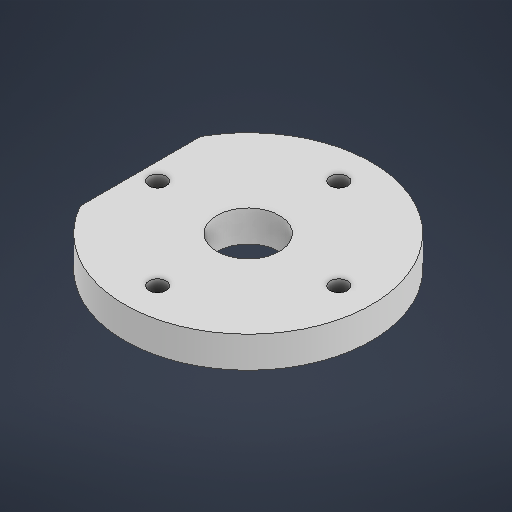
# Autodesk Inventor part: Adapter Plate
Saved by Autodesk Inventor 2025 (Build 290162000, 162)
## iProperties
Created: 2024-09-13
Part Number: Adapter Plate
Material: Generic
Document SubType Name: Modeling
Designer: mayhe
Density: 1 g/cm^3
Appearance: Default
Author: mayhe
Autodesk Inventor part; units mm, degrees
ref_plane "YZ Plane" through (0, 0, 0) normal (1, 0, 0) x (0, 1, 0)
ref_plane "XZ Plane" through (0, 0, 0) normal (0, 1, 0) x (-1, 0, 0)
ref_plane "XY Plane" through (0, 0, 0) normal (0, 0, 1) x (1, 0, 0)
sketch "Sketch1" plane through (0, 0, 0) normal (0, 1, 0) x (-1, 0, 0)
  circle A0 centre (0, 0) radius 39.5
  circle A1 centre (0, 0) radius 10
  circle A2 centre (0, 0) radius 29
  circle A3 centre (29, 0) radius 2.75
  circle A4 centre (0, 29) radius 2.75
  circle A5 centre (-29, 0) radius 2.75
  circle A6 centre (0, -29) radius 2.75
  dimension "d2" = 58
  dimension "d0" = 79
  dimension "d1" = 20
  dimension "d3" = 5.5
  dimension "d6" = 360
  constraints: 6 centre point, 3 coincident, 1 horizontal alignment, 11 other
  measures "d0" diameter of A0
  measures "d1" diameter of A1
  measures "d3" diameter of A3
extrude "Extrusion1" add sketch "Sketch1" along normal blind 10 contours A0 | A3 A2 A6 A5 A4
sketch "Sketch2" plane through (0, 0, 0) normal (0, -1, 0) x (1, 0, 0)
  circle A0 centre (0, -29) radius 2.75 projected
  circle A1 centre (0, 0) radius 29
  circle A2 centre (29, 0) radius 2.75 projected
  circle A3 centre (29, 0) radius 4
  circle A4 centre (0, 29) radius 4
  circle A5 centre (-29, 0) radius 4
  circle A6 centre (0, -29) radius 4
  line L0 (25, 2.3094) -> (29, 4.6188)
  line L1 (29, 4.6188) -> (33, 2.3094)
  line L2 (33, 2.3094) -> (33, -2.3094)
  line L3 (33, -2.3094) -> (29, -4.6188)
  line L4 (29, -4.6188) -> (25, -2.3094)
  line L5 (25, -2.3094) -> (25, 2.3094)
  line L6 (-4, -26.6906) -> (0, -24.3812)
  line L7 (0, -24.3812) -> (4, -26.6906)
  line L8 (4, -26.6906) -> (4, -31.3094)
  line L9 (4, -31.3094) -> (0, -33.6188)
  line L10 (0, -33.6188) -> (-4, -31.3094)
  line L11 (-4, -31.3094) -> (-4, -26.6906)
  line L12 (-33, 2.3094) -> (-29, 4.6188)
  line L13 (-29, 4.6188) -> (-25, 2.3094)
  line L14 (-25, 2.3094) -> (-25, -2.3094)
  line L15 (-25, -2.3094) -> (-29, -4.6188)
  line L16 (-29, -4.6188) -> (-33, -2.3094)
  line L17 (-33, -2.3094) -> (-33, 2.3094)
  line L18 (-4, 31.3094) -> (0, 33.6188)
  line L19 (0, 33.6188) -> (4, 31.3094)
  line L20 (4, 31.3094) -> (4, 26.6906)
  line L21 (4, 26.6906) -> (0, 24.3812)
  line L22 (0, 24.3812) -> (-4, 26.6906)
  line L23 (-4, 26.6906) -> (-4, 31.3094)
  circle A7 centre (0, 29) radius 2.75
  circle A8 centre (-29, 0) radius 2.75
  point P0 (25, 0)
  point P1 (-4, -29)
  point P2 (-33, 0)
  point P3 (-4, 29)
  dimension "d10" = 8
  dimension "d13" = 360
  constraints: 48 end point, 8 coincident, 4 horizontal alignment, 4 midpoint, 2 centre point, 1 point on line, 1 vertical alignment, 71 other
extrude "Extrusion2" cut sketch "Sketch2" against normal blind 4 contours A0 A1 A6 | A0 A1 A6 | A6 L7 L8 A1 | A1 L8 A6 | A6 L11 A1 | A1 L11 L6 A6 | L8 L9 A6 | A6 L6 L7 | A6 L10 L11 | L4 A3 A1 | A1 A3 L3 L4 | L9 L10 A6 | L15 L16 A5 A1 | A1 A5 L15 | A3 A1 A2 | A1 A2 A3 | L4 L5 A3 | A5 A1 A8 | A1 A8 A5 | A5 L14 L15 | A3 L2 L3 | L5 L0 A3 | L16 L17 A5 | A5 L13 L14 | A3 L1 L2 | L0 A1 A3 | L17 L12 A5 | A5 A1 L13 | A1 L0 L1 A3 | A5 L12 L13 A1 | L20 L21 A4 A1 | A1 A4 L20 | L23 A4 A1 | A1 A4 L22 L23 | A4 A1 A7 | A1 A7 A4 | A4 L19 L20 | L23 L18 A4 | L21 L22 A4 | A4 L18 L19
sketch "Sketch3" plane through (0, 10, 0) normal (0, 1, 0) x (1, 0, 0)
  line L0 (-34.5, 50.157) -> (-34.5, -49.8555)
  circle A0 centre (0, 0) radius 39.5 projected
  point P0 (-34.5, -19.2354)
  point P1 (-34.5, 19.2354)
  dimension "d18" = 5
  constraints: 2 end point, 1 vertical
  measures "d18" distance edge to line of A0 L0
extrude "Extrusion3" cut sketch "Sketch3" along normal through all both and the other way through all contours L0 A0 picked at (-35.5583, 3.956)
body "Solid1"
